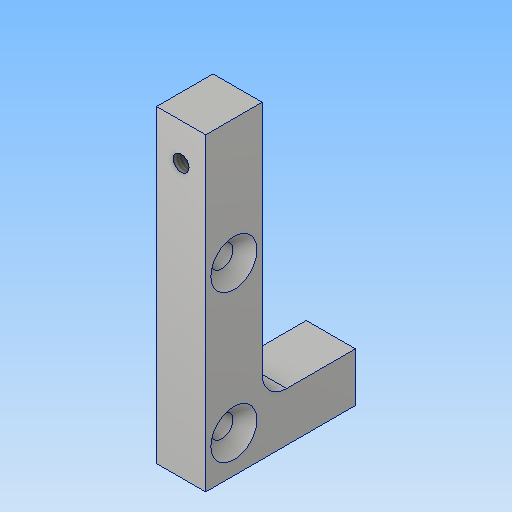
# Autodesk Inventor part: Pancake_Flexi Pipe Mount 2
Saved by Autodesk Inventor 2018.1 (Build 221171000, 171)
## iProperties
Created: 2019-02-26
Part Number: Pancake_Flexi Pipe Mount 2
Material: Aluminum 6061
Document SubType Name: Modeling
Designer: James
Density: 2.7 g/cm^3
Appearance: Aluminum - Flat
Mass: 23.1387 g
Surface Area: 41.0462 cm^2
Volume: 8.56988 cm^3
Author: James
Autodesk Inventor part; units mm, degrees
ref_plane "YZ Plane" through (0, 0, 0) normal (1, 0, 0) x (0, 1, 0)
ref_plane "XZ Plane" through (0, 0, 0) normal (0, 1, 0) x (-1, 0, 0)
ref_plane "XY Plane" through (0, 0, 0) normal (0, 0, 1) x (1, 0, 0)
sketch "Sketch1" plane through (0, 0, 0) normal (0, 0, 1) x (1, 0, 0)
  line L0 (0, 0) -> (10, 0)
  line L1 (10, 0) -> (10, 63)
  line L2 (10, 63) -> (0, 63)
  line L3 (0, 63) -> (0, 0)
  dimension "d0" = 10
  dimension "d1" = 63
  constraints: 8 end point, 2 parallel, 1 horizontal, 1 perpendicular
  measures "d0" distance of L0.start L0.end
  measures "d1" distance of L0.end L1.end
extrude "Extrusion1" add sketch "Sketch1" along normal blind 11.5
sketch "Sketch2" plane through (0, 0, 11.5) normal (0, 0, 1) x (1, 0, 0)
  line L0 (10, 63) -> (0, 63) projected
  line L1 (0, 0) -> (10, 0) projected
  point P0 (5, 55.5)
  point P1 (5, 63)
  dimension "d5" = 7.5
  dimension "d24" = 63
  constraints: 1 midpoint, 1 vertical alignment
  measures "d5" distance from line of L0 point (5, 55.5)
  measures "d24" distance between parallel lines of L1 L0
hole "Hole1" at (5, 55.5, 11.5) direction (0, 0, -1) diameter 3.242 end through all thread size "M4x0.7" class "6H" standard "ANSI Metric M Profile"
sketch "Sketch3" plane through (10, 0, 0) normal (1, 0, 0) x (0, 0, -1)
  line L0 (0, 63) -> (-11.5, 63) projected
  line L1 (0, 0) -> (-11.5, 0) projected
  point P0 (-5.75, 37.5)
  point P1 (-5.75, 7.5)
  point P2 (-5.75, 63)
  dimension "d16" = 7.5
  dimension "d25" = 30
  constraints: 2 vertical alignment, 1 midpoint
  measures "d16" distance from line of L1 point (-5.75, 7.5)
  measures "d25" distance of point (-5.75, 7.5) point (-5.75, 37.5)
hole "Hole2" at (10, 37.5, 5.75) at (10, 7.5, 5.75) direction (-1, 0, 0) diameter 4.5 end through all countersink diameter 9.4 countersink angle 90 clearance for "Flat Head Machine Screw" size "M4" standard "Ansi Metric M Profile"
sketch "Sketch4" plane through (0, 0, 0) normal (0, 0, -1) x (-1, 0, 0)
  point P0 (0, 0)
sketch "Sketch5" plane through (0, 0, 0) normal (0, 0, -1) x (-1, 0, 0)
  line L0 (0, 0) -> (-10, 0)
  line L1 (-10, 0) -> (-10, 10)
  line L2 (-10, 10) -> (0, 10)
  line L3 (0, 10) -> (0, 0)
  line L4 (-10, 0) -> (-10, 63) projected
  dimension "d26" = 10
  constraints: 8 end point, 2 parallel, 1 horizontal, 1 perpendicular, 1 point on line
  measures "d26" distance of L0.end L1.end
extrude "Extrusion2" add sketch "Sketch5" along normal blind 19
sketch "Sketch6" plane through (0, 0, -19) normal (0, 0, -1) x (-1, 0, 0)
  line L0 (-10, 0) -> (0, 0) projected
  line L1 (0, 10) -> (-10, 10) projected
  circle A0 centre (-5, 55.5) radius 1.621 projected
  point P0 (-5, 4.5)
  point P1 (-5, 0)
  dimension "d31" = 51
  constraints: 1 midpoint, 1 vertical alignment
  measures "d31" distance of point (-5, 4.5) A0.centre
hole "Hole3" at (5, 4.5, -19) direction (0, 0, 1) diameter 3.242 depth 11.8 tip angle 118 thread size "M4x0.7" class "6H" standard "ANSI Metric M Profile"
fillet "Fillet1" radius 5 1 edges at (5, 10, 0)
body "Solid1"
